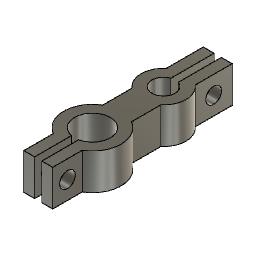
JRCNC0012 v8 (Autodesk Fusion 360 design; units mm, degrees)
Autodesk Fusion 360 part; units mm, degrees
note: some values were not read from the file. Set by a fixed rule: which sketch regions a step uses.
sketch "Sketch1" plane through (0, 0, 0) normal (0, 0, 1) x (1, 0, 0)
  circle A0 centre (0, 0) radius 4.064
  circle A1 centre (0, 0) radius 7.874
  circle A2 centre (0, -25) radius 10.06
  circle A3 centre (0, -25) radius 6.25
  line L0 (0, 0) -> (0, -25) construction
  line L1 (4.064, 0) -> (-4.064, 0)
  line L2 (-4.064, 0) -> (-4.064, -25)
  line L3 (-4.064, -25) -> (4.064, -25)
  line L4 (4.064, -25) -> (4.064, 0)
  line L5 (4.064, 0) -> (-4.064, -25) construction
  line L6 (-4.064, 0) -> (4.064, -25) construction
  line L7 (-1.27, 19.05) -> (1.27, 19.05)
  line L8 (1.27, 19.05) -> (1.27, -44.05)
  line L9 (1.27, -44.05) -> (-1.27, -44.05)
  line L10 (-1.27, -44.05) -> (-1.27, 19.05)
  line L11 (-1.27, 19.05) -> (1.27, -44.05) construction
  line L12 (1.27, 19.05) -> (-1.27, -44.05) construction
  line L13 (-5.08, 19.05) -> (5.08, 19.05)
  line L14 (5.08, 19.05) -> (5.08, -44.05)
  line L15 (5.08, -44.05) -> (-5.08, -44.05)
  line L16 (-5.08, -44.05) -> (-5.08, 19.05)
  line L17 (-5.08, 19.05) -> (5.08, -44.05) construction
  line L18 (5.08, 19.05) -> (-5.08, -44.05) construction
  point P0 (0, -12.5)
  point P1 (0, -12.5)
  point P2 (0, -12.5)
  dimension "d2" = 3.81
  dimension "d3" = 8.128
  dimension "d4" = 12.5
  dimension "d5" = 3.81
  dimension "d10" = 25
  dimension "d11" = 3.81
  dimension "d13" = 2.54
  dimension "d15" = 19.05
  constraint coincident A0.centre A1.centre
  constraint concentric A2 A3
  constraint vertical L0
  constraint coincident A2.centre A3.centre
  constraint horizontal L1
  constraint perpendicular L1 L2
  constraint parallel L1 L3
  constraint parallel L2 L4
  constraint coincident A0 L1.start
  constraint coincident L5 P2
  constraint coincident L6 P2
  constraint midpoint L0 P2
  constraint coincident A0.centre L1
  constraint horizontal L7
  constraint perpendicular L7 L8
  constraint parallel L7 L9
  constraint parallel L8 L10
  constraint coincident L11 P2
  constraint coincident L12 P2
  constraint coincident P2 P1
  constraint horizontal L13
  constraint perpendicular L13 L14
  constraint parallel L13 L15
  constraint parallel L14 L16
  constraint coincident L17 P2
  constraint coincident L18 P2
  constraint coincident L9.end L15
  measures "d2" distance of A0 A1
  measures "d3" diameter of A0
  measures "d4" diameter of A3
  measures "d5" distance of A2 A3
  measures "d10" distance of L1.start L3.end
  measures "d11" distance of L10 L16
  measures "d13" distance of L8 L10
  measures "d15" vertical distance of A2.centre L15.end
extrude "Extrude1" add sketch "Sketch1" along normal blind 12.7 contours A0 A1 L4 L8 | A0 A1 L4 L8 L14 | A0 A1 L8 L10 | A1 A2 L4 L8 | A1 A2 L4 L14 | A0 A1 L2 L10 L16 | A1 L8 L13 L14 | A0 A1 L2 L10 | A1 A2 L8 L10 | A1 L14 | A2 A3 L4 L8 | A2 A3 L4 L14 | A1 L10 L13 L16 | A1 A2 L2 L10 | A2 A3 L8 L10 | A2 A3 L14 | A1 A2 L2 L16 | A1 L16 | A2 A3 L2 L10 | A2 A3 L2 L16 | A2 L8 L14 L15 | A2 A3 L8 L14 | A2 A3 L16 | A2 A3 L10 L16 | A2 L10 L15 L16 picked at (-0.651, -6.5631) picked at (0.9887, -17.5551)
sketch "Sketch2" plane through (5.08, 0, 0) normal (1, 0, 0) x (0, 1, 0)
  line L0 (-44.05, 0) -> (-33.6832, 0)
  line L1 (-33.6832, 0) -> (-33.6832, 12.7)
  line L2 (-33.6832, 12.7) -> (-44.05, 12.7)
  line L3 (-44.05, 12.7) -> (-44.05, 0)
  line L4 (-38.8666, 12.7) -> (-38.8666, 0)
  point P0 (-38.8666, 6.35)
  constraint midpoint L2 L4.start
  constraint midpoint L0 L4.end
  constraint midpoint L4 P0
hole "Hole1" at (5.08, -38.8666, 6.35) direction (-1, 0, 0) diameter 5.5118 depth 40.64 tip angle 180
sketch "Sketch3" plane through (5.08, 0, 0) normal (1, 0, 0) x (0, 1, 0)
  line L0 (6.0161, 0) -> (19.05, 0)
  line L1 (19.05, 0) -> (19.05, 12.7)
  line L2 (19.05, 12.7) -> (6.0161, 12.7)
  line L3 (6.0161, 12.7) -> (6.0161, 0)
  line L4 (12.5331, 12.7) -> (12.5331, 0)
  point P0 (12.5331, 6.35)
  constraint midpoint L2 L4.start
  constraint midpoint L0 L4.end
  constraint midpoint L4 P0
hole "Hole2" at (5.08, 12.5331, 6.35) direction (-1, 0, 0) diameter 5.5118 depth 40.64 tip angle 180
